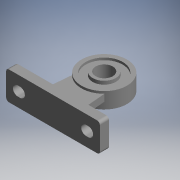
# Autodesk Inventor part: PDRHN30_b
Saved by Autodesk Inventor 2017.3 (Build 213256000, 256)
## iProperties
Part Number: PDRHN30_b
Material: Generic
Catalog Web Link: www.cadenas.de
Description: PDRH,PDRHN_body-Ball Bearing Units -High-Centered Pillow Type-
Vendor: MISUMI
Document SubType Name: Modeling
Designer: partserver
Manufacturer: MISUMI
Mass: 268.59 g
Surface Area: 523.173 cm^2
Volume: 268.59 cm^3
Density: 1 g/cm^3
Appearance: PSOLRGB-175-175-175
Category: PARTsolutions
Company: MISUMI
Title: PDRHN30
Author: Cadenas PARTsolutions
Comments: Ball Bearing Units -High-Centered Pillow Type-
PSOL_IDENT_0: {$CADENAS_DATA\23d-libs\misumi\metric\12_bearing_holders\pdrh\pdrh_body.prj},167 {VTYP=3D},{NB=PDRHN
PSOL_IDENT_1: 30_b},{LINA=PDRHN30},{NN=PDRH,PDRHN_body},{DATE=11.12.2019 10:04:59},{GEOMDATE=02.12.2019 07:12:02},
PSOL_IDENT_2: {VERSION=},{LINEID=60},{WBVAR=TS},{WBNUMERIC=}  {NB=PDRHN30_b},{LINA=PDRHN30},{KT=DUMMY},{PN=PDRHN30
PSOL_IDENT_3: },{TYPE=PDRHN},{MATH=Cast Iron Class No.30},{MATB=52100 Bearing Steel},{MATRS=Nitrile Rubber},{MATSS=
PSOL_IDENT_4: 4137 Alloy Steel},{PRECISION=JIS B 1558/JIS B 1514/JIS B 1559},{OT=-15 ~+100},{TS=2},{TSALG='1','Lub
PSOL_IDENT_5: rication Type' , '2','Oil-Free Type'},{D=30},{JIS=UC206D1},{H=90},{L=165},{L1=120},{A=50},{DD1=21},{
PSOL_IDENT_6: DD=17},{TT=16},{H1=130},{B=38.1},{S=15.9},{CR=19.5},{COR=11.30},{M1=M6x0.75},{MD=6},{MPITCH=0.75},{M
PSOL_IDENT_7: L=8},{MASS=1800},{RLD1=80},{RLD2=65},{RLD3=40.8},{LD1=28},{LD2=4.0},{LD3=2},{G1=28.5},{G2=12.0},{G3=
PSOL_IDENT_8: 50},{R1=11},{R2=5},{NCL=1.9},{KCL=17.2}
NB: PDRHN30_b
NN: PDRH,PDRHN_body
NT: Ball Bearing Units -High-Centered Pillow Type-
NBSYN: $PN._b
LINA: PDRHN30
CATALOG: Misumi
PN: PDRHN30
TYPE: PDRHN
MATH: Cast Iron Class No.30
MATB: 52100 Bearing Steel
MATRS: Nitrile Rubber
MATSS: 4137 Alloy Steel
PRECISION: JIS B 1558/JIS B 1514/JIS B 1559
OT: -15 ~+100
TS: Oil-Free Type
D: 30
JIS: UC206D1
H: 90
L: 165
L1: 120
A: 50
DD1: 21
DD: 17
TT: 16
H1: 130
B: 38.1
S: 15.9
CR: 19.5
COR: 11.3
M1: M6x0.75
MASS: 1800
SUPPLIER: MISUMI
ARTICLENO: PDRHN30_b
BOMINFO: PDRHN30
CREATOR: CADENAS GmbH
Autodesk Inventor part; units mm, degrees
sketch "_____3" plane through (0, 0, -14) normal (0, 0, 1) x (1, 0, 0)
  line L0 (-42.59827, 16) -> (42.59827, 16)
  arc A0 (31.640128, 26.041287) -> (42.59827, 16) centre (42.59827, 27) ccw
  line L1 (31.640128, 26.041287) -> (28.5, 61.933116)
  arc A1 (28.5, 61.933116) -> (-28.5, 61.933116) centre (0, 90) ccw
  line L2 (-28.5, 61.933116) -> (-31.640128, 26.041287)
  arc A2 (-42.59827, 16) -> (-31.640128, 26.041287) centre (-42.59827, 27) ccw
  constraints: 6 end point, 6 point on circle, 3 centre point
extrude "Extrusion1" add sketch "_____3" along normal blind 39
sketch "_____8" plane through (0, 0, 0) normal (1, 0, 0) x (0, 0, -1)
  line L0 (-25, 52.45256) -> (-25, 16)
  line L1 (-25, 16) -> (-14, 50)
  line L2 (-14, 50) -> (-14, 52.45256)
  line L3 (-14, 52.45256) -> (-25, 52.45256)
  constraints: 8 end point
extrude "Extrusion2" cut sketch "_____8" along normal mid plane 24
sketch "_____9" plane through (0, 0, 0) normal (1, 0, 0) x (0, 0, -1)
  line L0 (-14, 90) -> (-25, 90)
  line L1 (-25, 90) -> (-25, 130)
  line L2 (-25, 130) -> (-14, 130)
  line L3 (-14, 130) -> (-14, 90)
  line L4 (-14, 90) -> (-25, 90)
  constraints: 10 end point
revolve "Revolution1" cut sketch "_____9" angle 360 about axis through (0, 90, 14) along (0, 0, -1)
sketch "_____5" plane through (0, 0, 25) normal (0, 0, 1) x (1, 0, 0)
  line L0 (-50, 90) -> (-50, 0)
  line L1 (-50, 0) -> (50, 0)
  line L2 (50, 0) -> (50, 90)
  line L3 (50, 90) -> (40, 90)
  arc A0 (6, 50.45256) -> (40, 90) centre (0, 90) ccw
  line L4 (6, 50.45256) -> (6, 16)
  line L5 (6, 16) -> (-6, 16)
  line L6 (-6, 16) -> (-6, 50.45256)
  arc A1 (-40, 90) -> (-6, 50.45256) centre (0, 90) ccw
  line L7 (-40, 90) -> (-50, 90)
  constraints: 16 end point, 4 point on circle, 2 centre point
extrude "Extrusion3" cut sketch "_____5" against normal blind 23
sketch "_____6" plane through (0, 0, -14) normal (0, 0, 1) x (1, 0, 0)
  line L0 (-50, 90) -> (-50, 0)
  line L1 (-50, 0) -> (50, 0)
  line L2 (50, 0) -> (50, 90)
  line L3 (50, 90) -> (40, 90)
  arc A0 (-40, 90) -> (40, 90) centre (0, 90) ccw
  line L4 (-40, 90) -> (-50, 90)
  constraints: 10 end point, 2 point on circle, 1 centre point
extrude "Extrusion4" cut sketch "_____6" along normal blind 4
sketch "_____4" plane through (0, 0, 0) normal (0, 1, 0) x (1, 0, 0)
  line L0 (-82.5, 20) -> (-82.5, -20)
  arc A0 (-82.5, -20) -> (-77.5, -25) centre (-77.5, -20) ccw
  line L1 (-77.5, -25) -> (77.5, -25)
  arc A1 (77.5, -25) -> (82.5, -20) centre (77.5, -20) ccw
  line L2 (82.5, -20) -> (82.5, 20)
  arc A2 (82.5, 20) -> (77.5, 25) centre (77.5, 20) ccw
  line L3 (77.5, 25) -> (-77.5, 25)
  arc A3 (-77.5, 25) -> (-82.5, 20) centre (-77.5, 20) ccw
  constraints: 8 end point, 8 point on circle, 4 centre point
extrude "Extrusion5" add sketch "_____4" along normal blind 16
sketch "_____7" plane through (0, 0, 0) normal (0, 1, 0) x (1, 0, 0)
  arc A0 (58, 8.5) -> (58, -8.5) centre (58, 0) ccw
  line L0 (58, -8.5) -> (62, -8.5)
  arc A1 (62, -8.5) -> (62, 8.5) centre (62, 0) ccw
  line L1 (62, 8.5) -> (58, 8.5)
  constraints: 4 end point, 4 point on circle, 2 centre point
extrude "Extrusion6" cut sketch "_____7" along normal blind 16
sketch "_____10" plane through (0, 0, 0) normal (0, 1, 0) x (1, 0, 0)
  arc A0 (-62, 8.5) -> (-62, -8.5) centre (-62, 0) ccw
  line L0 (-62, -8.5) -> (-58, -8.5)
  arc A1 (-58, -8.5) -> (-58, 8.5) centre (-58, 0) ccw
  line L1 (-58, 8.5) -> (-62, 8.5)
  constraints: 4 end point, 4 point on circle, 2 centre point
extrude "Extrusion7" cut sketch "_____10" along normal blind 16
sketch "_____11" plane through (0, 0, 0) normal (1, 0, 0) x (0, 0, -1)
  line L0 (-10, 90) -> (-14, 90)
  line L1 (-14, 90) -> (-14, 122.5)
  line L2 (-14, 122.5) -> (-10, 122.5)
  line L3 (-10, 122.5) -> (-10, 90)
  line L4 (-10, 90) -> (-14, 90)
  constraints: 10 end point
revolve "Revolution2" cut sketch "_____11" angle 360 about axis through (0, 90, 10) along (0, 0, -1)
sketch "Sketch10" plane through (0, 90, -14) normal (0, 0, -1) x (-1, 0, 0)
  point P0 (0, 0)
hole "Hole1" at (0, 90, -14) direction (0, 0, 1) diameter 65 depth 4
sketch "_____13" plane through (0, 0, 0) normal (1, 0, 0) x (0, 0, -1)
  line L0 (15.9, 90) -> (-22.2, 90)
  line L1 (-22.2, 90) -> (-22.2, 110.4)
  line L2 (-22.2, 110.4) -> (15.9, 110.4)
  line L3 (15.9, 110.4) -> (15.9, 90)
  line L4 (15.9, 90) -> (-22.2, 90)
  constraints: 10 end point
revolve "Revolution3" add sketch "_____13" angle 360 about axis through (0, 90, -15.9) along (0, 0, -1)
sketch "Sketch12" plane through (0, 90, -15.9) normal (0, 0, -1) x (-1, 0, 0)
  point P0 (0, 0)
hole "Hole2" at (0, 90, -15.9) direction (0, 0, 1) diameter 30 depth 38.1
sketch "_____15" plane through (0, 0, 17.2) normal (0, 0, 1) x (1, 0, 0)
  line L0 (0, 90) -> (0, 110.4)
  line L1 (0, 110.4) -> (3, 110.4)
  line L2 (3, 110.4) -> (2.594, 109.994)
  line L3 (2.594, 109.994) -> (2.594, 90)
  line L4 (2.594, 90) -> (0, 90)
  line L5 (0, 90) -> (0, 110.4)
  constraints: 12 end point
revolve "Revolution4" cut sketch "_____15" angle 360 about axis through (0, 90, 17.2) along (0, -1, 0)
thread "Thread1" size "M6x0.75" class "6H" standard "ISO Metric profile" length 4.994
sketch "_____16" plane through (0, 0, 17.2) normal (0, 0, 1) x (1, 0, 0)
  line L0 (0, 90) -> (-17.666918, 79.8)
  line L1 (-17.666918, 79.8) -> (-19.166918, 82.398076)
  line L2 (-19.166918, 82.398076) -> (-18.612312, 82.24947)
  line L3 (-18.612312, 82.24947) -> (-1.297, 92.24647)
  line L4 (-1.297, 92.24647) -> (0, 90)
  line L5 (0, 90) -> (-17.666918, 79.8)
  constraints: 12 end point
revolve "Revolution5" cut sketch "_____16" angle 360 about axis through (0, 90, 17.2) along (0.8660254, 0.5, 0)
thread "Thread2" size "M6x0.75" class "6H" standard "ISO Metric profile" length 4.994
ref_plane "CP1_XY" through (0, 105, 17.2) normal (0, 1, 0) x (1, 0, 0)
ref_plane "CP1_YZ" through (0, 105, 17.2) normal (1, 0, 0) x (0, 0, -1)
ref_plane "CP1_ZX" through (0, 105, 17.2) normal (0, 0, -1) x (0, 1, 0)
ref_plane "CP2_XY" through (-12.990381, 82.5, 17.2) normal (-0.8660254, -0.5, 0) x (-0.5, 0.8660254, 0)
ref_plane "CP2_YZ" through (-12.990381, 82.5, 17.2) normal (-0.5, 0.8660254, 0) x (0, 0, -1)
ref_plane "CP2_ZX" through (-12.990381, 82.5, 17.2) normal (0, 0, -1) x (-0.8660254, -0.5, 0)
body "Solid1"
